Autodesk Inventor part; units mm, degrees
(part 4 of 7)
  line L2571 (-175.0784, 15.5559) -> (-174.9573, 15.634)
  line L2572 (-174.9573, 15.634) -> (-174.8636, 15.7434)
  line L2573 (-174.8636, 15.7434) -> (-174.7994, 15.9277)
  line L2574 (-174.7994, 15.9277) -> (-174.7854, 16.1223)
  line L2575 (-174.7854, 16.1223) -> (-174.7958, 16.3635)
  line L2576 (-174.7958, 16.3635) -> (-174.8284, 16.6028)
  line L2577 (-174.8284, 16.6028) -> (-173.8558, 16.7629)
  line L2578 (-173.8558, 16.7629) -> (-173.7931, 16.4252)
  line L2579 (-173.7931, 16.4252) -> (-173.7637, 16.0838)
  line L2580 (-173.7637, 16.0838) -> (-173.7676, 15.7411)
  line L2581 (-173.7676, 15.7411) -> (-173.805, 15.3997)
  line L2582 (-173.805, 15.3997) -> (-173.8689, 15.171)
  line L2583 (-173.8689, 15.171) -> (-173.9746, 14.9609)
  line L2584 (-173.9746, 14.9609) -> (-174.1185, 14.7748)
  line L2585 (-174.1185, 14.7748) -> (-174.2972, 14.6184)
  line L2586 (-174.2972, 14.6184) -> (-174.4447, 14.5464)
  line L2587 (-174.4447, 14.5464) -> (-174.5992, 14.4921)
  line L2588 (-174.5992, 14.4921) -> (-174.7588, 14.4561)
  line L2589 (-174.7588, 14.4561) -> (-174.9222, 14.4387)
  line L2590 (-174.9222, 14.4387) -> (-175.2129, 14.4186)
  line L2591 (-175.2129, 14.4186) -> (-175.5042, 14.4075)
  line L2592 (-175.5042, 14.4075) -> (-179.4729, 14.4075)
  line L2593 (-179.4729, 14.4075) -> (-179.4729, 13.5989)
  line L2594 (-179.4729, 13.5989) -> (-180.3245, 13.5989)
  line L2595 (-180.3245, 13.5989) -> (-180.3245, 14.4075)
  line L2596 (-180.3245, 14.4075) -> (-181.93, 14.4075)
  line L2597 (-181.93, 14.4075) -> (-182.5901, 15.4973)
  line L2598 (-182.5901, 15.4973) -> (-180.3245, 15.4973)
  line L2599 (-173.844, -41.0652) -> (-173.844, -42.1668)
  line L2600 (-173.844, -42.1668) -> (-180.3245, -42.1668)
  line L2601 (-180.3245, -42.1668) -> (-180.3245, -41.0652)
  line L2602 (-180.3245, -41.0652) -> (-173.844, -41.0652)
  line L2603 (-173.844, -38.3464) -> (-173.844, -39.4441)
  line L2604 (-173.844, -39.4441) -> (-182.7933, -39.4441)
  line L2605 (-182.7933, -39.4441) -> (-182.7933, -38.3464)
  line L2606 (-182.7933, -38.3464) -> (-173.844, -38.3464)
  line L2607 (-179.5823, -48.073) -> (-179.7843, -47.8837)
  line L2608 (-179.7843, -47.8837) -> (-179.964, -47.674)
  line L2609 (-179.964, -47.674) -> (-180.1198, -47.4461)
  line L2610 (-180.1198, -47.4461) -> (-180.2503, -47.2019)
  line L2611 (-180.2503, -47.2019) -> (-180.3496, -46.9447)
  line L2612 (-180.3496, -46.9447) -> (-180.4202, -46.6789)
  line L2613 (-180.4202, -46.6789) -> (-180.4614, -46.4071)
  line L2614 (-180.4614, -46.4071) -> (-180.4729, -46.1316)
  line L2615 (-180.4729, -46.1316) -> (-180.4545, -45.7939)
  line L2616 (-180.4545, -45.7939) -> (-180.4026, -45.4597)
  line L2617 (-180.4026, -45.4597) -> (-180.3417, -45.2394)
  line L2618 (-180.3417, -45.2394) -> (-180.2591, -45.0268)
  line L2619 (-180.2591, -45.0268) -> (-180.1555, -44.8237)
  line L2620 (-180.1555, -44.8237) -> (-180.0315, -44.6316)
  line L2621 (-180.0315, -44.6316) -> (-179.9006, -44.4735)
  line L2622 (-179.9006, -44.4735) -> (-179.7507, -44.3344)
  line L2623 (-179.7507, -44.3344) -> (-179.5841, -44.216)
  line L2624 (-179.5841, -44.216) -> (-179.4026, -44.1199)
  line L2625 (-179.4026, -44.1199) -> (-179.0103, -43.9893)
  line L2626 (-179.0103, -43.9893) -> (-178.6019, -43.9246)
  line L2627 (-178.6019, -43.9246) -> (-178.3932, -43.9046)
  line L2628 (-178.3932, -43.9046) -> (-178.1839, -43.8933)
  line L2629 (-178.1839, -43.8933) -> (-173.844, -43.8933)
  line L2630 (-173.844, -43.8933) -> (-173.844, -44.991)
  line L2631 (-173.844, -44.991) -> (-177.9534, -44.991)
  line L2632 (-177.9534, -44.991) -> (-178.2064, -44.9949)
  line L2633 (-178.2064, -44.9949) -> (-178.456, -45.0299)
  line L2634 (-178.456, -45.0299) -> (-178.6994, -45.0951)
  line L2635 (-178.6994, -45.0951) -> (-178.9339, -45.1902)
  line L2636 (-178.9339, -45.1902) -> (-179.0477, -45.262)
  line L2637 (-179.0477, -45.262) -> (-179.1526, -45.3464)
  line L2638 (-179.1526, -45.3464) -> (-179.3167, -45.5457)
  line L2639 (-179.3167, -45.5457) -> (-179.4339, -45.78)
  line L2640 (-179.4339, -45.78) -> (-179.5042, -46.0496)
  line L2641 (-179.5042, -46.0496) -> (-179.5275, -46.3227)
  line L2642 (-179.5275, -46.3227) -> (-179.512, -46.5964)
  line L2643 (-179.512, -46.5964) -> (-179.4618, -46.8331)
  line L2644 (-179.4618, -46.8331) -> (-179.3818, -47.0603)
  line L2645 (-179.3818, -47.0603) -> (-179.2731, -47.2753)
  line L2646 (-179.2731, -47.2753) -> (-179.137, -47.4753)
  line L2647 (-179.137, -47.4753) -> (-178.9754, -47.6411)
  line L2648 (-178.9754, -47.6411) -> (-178.7933, -47.7839)
  line L2649 (-178.7933, -47.7839) -> (-178.4433, -47.939)
  line L2650 (-178.4433, -47.939) -> (-178.0706, -48.0261)
  line L2651 (-178.0706, -48.0261) -> (-177.7316, -48.0626)
  line L2652 (-177.7316, -48.0626) -> (-177.3909, -48.073)
  line L2653 (-177.3909, -48.073) -> (-173.844, -48.073)
  line L2654 (-173.844, -48.073) -> (-173.844, -49.1707)
  line L2655 (-173.844, -49.1707) -> (-182.7933, -49.1707)
  line L2656 (-182.7933, -49.1707) -> (-182.7933, -48.073)
  line L2657 (-182.7933, -48.073) -> (-179.5823, -48.073)
  line L2658 (-180.4651, 4.47) -> (-180.4377, 4.7226)
  line L2659 (-180.4377, 4.7226) -> (-180.3791, 4.9689)
  line L2660 (-180.3791, 4.9689) -> (-180.2903, 5.2059)
  line L2661 (-180.2903, 5.2059) -> (-180.1722, 5.4309)
  line L2662 (-180.1722, 5.4309) -> (-179.9946, 5.661)
  line L2663 (-179.9946, 5.661) -> (-179.7797, 5.8532)
  line L2664 (-179.7797, 5.8532) -> (-179.5336, 6.0032)
  line L2665 (-179.5336, 6.0032) -> (-179.262, 6.1067)
  line L2666 (-179.262, 6.1067) -> (-179.0241, 6.167)
  line L2667 (-179.0241, 6.167) -> (-178.7826, 6.2087)
  line L2668 (-178.7826, 6.2087) -> (-178.5386, 6.2316)
  line L2669 (-178.5386, 6.2316) -> (-178.2933, 6.2356)
  line L2670 (-178.2933, 6.2356) -> (-173.844, 6.2356)
  line L2671 (-173.844, 6.2356) -> (-173.844, 5.1458)
  line L2672 (-173.844, 5.1458) -> (-177.9261, 5.1458)
  line L2673 (-177.9261, 5.1458) -> (-178.3184, 5.1359)
  line L2674 (-178.3184, 5.1359) -> (-178.7073, 5.0833)
  line L2675 (-178.7073, 5.0833) -> (-178.899, 5.0286)
  line L2676 (-178.899, 5.0286) -> (-179.0727, 4.9355)
  line L2677 (-179.0727, 4.9355) -> (-179.223, 4.808)
  line L2678 (-179.223, 4.808) -> (-179.344, 4.6497)
  line L2679 (-179.344, 4.6497) -> (-179.4364, 4.456)
  line L2680 (-179.4364, 4.456) -> (-179.4957, 4.2513)
  line L2681 (-179.4957, 4.2513) -> (-179.5212, 4.0398)
  line L2682 (-179.5212, 4.0398) -> (-179.512, 3.8254)
  line L2683 (-179.512, 3.8254) -> (-179.4814, 3.6006)
  line L2684 (-179.4814, 3.6006) -> (-179.4175, 3.3871)
  line L2685 (-179.4175, 3.3871) -> (-179.3228, 3.1881)
  line L2686 (-179.3228, 3.1881) -> (-179.1998, 3.0065)
  line L2687 (-179.1998, 3.0065) -> (-179.0509, 2.8455)
  line L2688 (-179.0509, 2.8455) -> (-178.8784, 2.7082)
  line L2689 (-178.8784, 2.7082) -> (-178.685, 2.5976)
  line L2690 (-178.685, 2.5976) -> (-178.4729, 2.5168)
  line L2691 (-178.4729, 2.5168) -> (-178.0457, 2.427)
  line L2692 (-178.0457, 2.427) -> (-177.6097, 2.4036)
  line L2693 (-177.6097, 2.4036) -> (-173.844, 2.4036)
  line L2694 (-173.844, 2.4036) -> (-173.844, 1.3059)
  line L2695 (-173.844, 1.3059) -> (-178.055, 1.3059)
  line L2696 (-178.055, 1.3059) -> (-178.3774, 1.2926)
  line L2697 (-178.3774, 1.2926) -> (-178.6956, 1.2395)
  line L2698 (-178.6956, 1.2395) -> (-178.9495, 1.1536)
  line L2699 (-178.9495, 1.1536) -> (-179.1526, 1.0364)
  line L2700 (-179.1526, 1.0364) -> (-179.283, 0.9168)
  line L2701 (-179.283, 0.9168) -> (-179.3855, 0.7748)
  line L2702 (-179.3855, 0.7748) -> (-179.4576, 0.6152)
  line L2703 (-179.4576, 0.6152) -> (-179.4964, 0.4426)
  line L2704 (-179.4964, 0.4426) -> (-179.5196, 0.088)
  line L2705 (-179.5196, 0.088) -> (-179.4659, -0.259)
  line L2706 (-179.4659, -0.259) -> (-179.3386, -0.5863)
  line L2707 (-179.3386, -0.5863) -> (-179.1409, -0.8816)
  line L2708 (-179.1409, -0.8816) -> (-179.0146, -1.0038)
  line L2709 (-179.0146, -1.0038) -> (-178.8751, -1.1096)
  line L2710 (-178.8751, -1.1096) -> (-178.724, -1.1982)
  line L2711 (-178.724, -1.1982) -> (-178.5628, -1.2683)
  line L2712 (-178.5628, -1.2683) -> (-178.0997, -1.384)
  line L2713 (-178.0997, -1.384) -> (-177.6253, -1.4363)
  line L2714 (-177.6253, -1.4363) -> (-177.2073, -1.448)
  line L2715 (-177.2073, -1.448) -> (-173.844, -1.448)
  line L2716 (-173.844, -1.448) -> (-173.844, -2.5457)
  line L2717 (-173.844, -2.5457) -> (-180.3245, -2.5457)
  line L2718 (-180.3245, -2.5457) -> (-180.3245, -1.5613)
  line L2719 (-180.3245, -1.5613) -> (-179.4183, -1.5613)
  line L2720 (-179.4183, -1.5613) -> (-179.6251, -1.4136)
  line L2721 (-179.6251, -1.4136) -> (-179.8124, -1.2453)
  line L2722 (-179.8124, -1.2453) -> (-179.9787, -1.0583)
  line L2723 (-179.9787, -1.0583) -> (-180.123, -0.8546)
  line L2724 (-180.123, -0.8546) -> (-180.2438, -0.6362)
  line L2725 (-180.2438, -0.6362) -> (-180.34, -0.4051)
  line L2726 (-180.34, -0.4051) -> (-180.4103, -0.1633)
  line L2727 (-180.4103, -0.1633) -> (-180.4534, 0.0872)
  line L2728 (-180.4534, 0.0872) -> (-180.4717, 0.3305)
  line L2729 (-180.4717, 0.3305) -> (-180.4686, 0.5739)
  line L2730 (-180.4686, 0.5739) -> (-180.4443, 0.8162)
  line L2731 (-180.4443, 0.8162) -> (-180.3987, 1.0559)
  line L2732 (-180.3987, 1.0559) -> (-180.305, 1.3372)
  line L2733 (-180.305, 1.3372) -> (-180.213, 1.5188)
  line L2734 (-180.213, 1.5188) -> (-180.1001, 1.6874)
  line L2735 (-180.1001, 1.6874) -> (-179.9675, 1.8409)
  line L2736 (-179.9675, 1.8409) -> (-179.8167, 1.9778)
  line L2737 (-179.8167, 1.9778) -> (-179.5867, 2.1241)
  line L2738 (-179.5867, 2.1241) -> (-179.3362, 2.2317)
  line L2739 (-179.3362, 2.2317) -> (-179.5865, 2.4154)
  line L2740 (-179.5865, 2.4154) -> (-179.8132, 2.6259)
  line L2741 (-179.8132, 2.6259) -> (-180.0144, 2.861)
  line L2742 (-180.0144, 2.861) -> (-180.1878, 3.1184)
  line L2743 (-180.1878, 3.1184) -> (-180.2864, 3.3111)
  line L2744 (-180.2864, 3.3111) -> (-180.364, 3.5125)
  line L2745 (-180.364, 3.5125) -> (-180.4198, 3.721)
  line L2746 (-180.4198, 3.721) -> (-180.4534, 3.9348)
  line L2747 (-180.4534, 3.9348) -> (-180.4724, 4.2021)
  line L2748 (-180.4724, 4.2021) -> (-180.4651, 4.47)
  line L2749 (-182.7854, -53.6121) -> (-182.7482, -52.9791)
  line L2750 (-182.7482, -52.9791) -> (-182.6409, -52.3543)
  line L2751 (-182.6409, -52.3543) -> (-182.5792, -52.146)
  line L2752 (-182.5792, -52.146) -> (-182.4996, -51.9443)
  line L2753 (-182.4996, -51.9443) -> (-182.4029, -51.7503)
  line L2754 (-182.4029, -51.7503) -> (-182.2894, -51.5652)
  line L2755 (-182.2894, -51.5652) -> (-182.0536, -51.2911)
  line L2756 (-182.0536, -51.2911) -> (-181.7801, -51.0579)
  line L2757 (-181.7801, -51.0579) -> (-181.4742, -50.8694)
  line L2758 (-181.4742, -50.8694) -> (-181.1409, -50.7293)
  line L2759 (-181.1409, -50.7293) -> (-180.8639, -50.6516)
  line L2760 (-180.8639, -50.6516) -> (-180.5826, -50.6009)
  line L2761 (-180.5826, -50.6009) -> (-180.2991, -50.5772)
  line L2762 (-180.2991, -50.5772) -> (-180.0153, -50.5802)
  line L2763 (-180.0153, -50.5802) -> (-179.733, -50.6099)
  line L2764 (-179.733, -50.6099) -> (-179.4541, -50.6663)
  line L2765 (-179.4541, -50.6663) -> (-179.1806, -50.749)
  line L2766 (-179.1806, -50.749) -> (-178.9144, -50.8582)
  line L2767 (-178.9144, -50.8582) -> (-178.6835, -50.9871)
  line L2768 (-178.6835, -50.9871) -> (-178.4675, -51.1383)
  line L2769 (-178.4675, -51.1383) -> (-178.2679, -51.3106)
  line L2770 (-178.2679, -51.3106) -> (-178.0862, -51.5027)
  line L2771 (-178.0862, -51.5027) -> (-177.9551, -51.6922)
  line L2772 (-177.9551, -51.6922) -> (-177.8432, -51.8931)
  line L2773 (-177.8432, -51.8931) -> (-177.7513, -52.1038)
  line L2774 (-177.7513, -52.1038) -> (-177.68, -52.323)
  line L2775 (-177.68, -52.323) -> (-177.5868, -52.7182)
  line L2776 (-177.5868, -52.7182) -> (-177.5224, -53.1185)
  line L2777 (-177.5224, -53.1185) -> (-177.487, -53.5225)
  line L2778 (-177.487, -53.5225) -> (-177.4808, -53.9285)
  line L2779 (-177.4808, -53.9285) -> (-177.4808, -56.2214)
  line L2780 (-177.4808, -56.2214) -> (-173.844, -56.2214)
  line L2781 (-173.844, -56.2214) -> (-173.844, -57.405)
  line L2782 (-173.844, -57.405) -> (-182.7933, -57.405)
  line L2783 (-182.7933, -57.405) -> (-182.7933, -54.03)
  line L2784 (-182.7933, -54.03) -> (-182.7854, -53.6121)
  line L2785 (-173.844, -6.9402) -> (-173.844, -8.0418)
  line L2786 (-173.844, -8.0418) -> (-180.3245, -8.0418)
  line L2787 (-180.3245, -8.0418) -> (-180.3245, -6.9402)
  line L2788 (-180.3245, -6.9402) -> (-173.844, -6.9402)
  line L2789 (-173.844, -4.2214) -> (-173.844, -5.3191)
  line L2790 (-173.844, -5.3191) -> (-182.7933, -5.3191)
  line L2791 (-182.7933, -5.3191) -> (-182.7933, -4.2214)
  line L2792 (-182.7933, -4.2214) -> (-173.844, -4.2214)
  line L2793 (-173.844, -35.5652) -> (-173.844, -36.6668)
  line L2794 (-173.844, -36.6668) -> (-180.3245, -36.6668)
  line L2795 (-180.3245, -36.6668) -> (-180.3245, -35.5652)
  line L2796 (-180.3245, -35.5652) -> (-173.844, -35.5652)
  line L2797 (-180.4495, 44.1145) -> (-180.3987, 44.3381)
  line L2798 (-180.3987, 44.3381) -> (-180.326, 44.555)
  line L2799 (-180.326, 44.555) -> (-180.232, 44.7635)
  line L2800 (-180.232, 44.7635) -> (-180.1175, 44.9621)
  line L2801 (-180.1175, 44.9621) -> (-179.0979, 44.5871)
  line L2802 (-179.0979, 44.5871) -> (-179.2175, 44.3584)
  line L2803 (-179.2175, 44.3584) -> (-179.2959, 44.1144)
  line L2804 (-179.2959, 44.1144) -> (-179.332, 43.8607)
  line L2805 (-179.332, 43.8607) -> (-179.3245, 43.6028)
  line L2806 (-179.3245, 43.6028) -> (-179.2233, 43.3038)
  line L2807 (-179.2233, 43.3038) -> (-179.0473, 43.0488)
  line L2808 (-179.0473, 43.0488) -> (-178.8087, 42.851)
  line L2809 (-178.8087, 42.851) -> (-178.5198, 42.7239)
  line L2810 (-178.5198, 42.7239) -> (-178.2054, 42.6419)
  line L2811 (-178.2054, 42.6419) -> (-177.8861, 42.5838)
  line L2812 (-177.8861, 42.5838) -> (-177.5634, 42.5499)
  line L2813 (-177.5634, 42.5499) -> (-177.2386, 42.5403)
  line L2814 (-177.2386, 42.5403) -> (-173.844, 42.5403)
  line L2815 (-173.844, 42.5403) -> (-173.844, 41.4426)
  line L2816 (-173.844, 41.4426) -> (-180.3245, 41.4426)
  line L2817 (-180.3245, 41.4426) -> (-180.3245, 42.4309)
  line L2818 (-180.3245, 42.4309) -> (-179.344, 42.4309)
  line L2819 (-179.344, 42.4309) -> (-179.7479, 42.671)
  line L2820 (-179.7479, 42.671) -> (-180.1136, 42.9661)
  line L2821 (-180.1136, 42.9661) -> (-180.2676, 43.1524)
  line L2822 (-180.2676, 43.1524) -> (-180.3807, 43.3634)
  line L2823 (-180.3807, 43.3634) -> (-180.4501, 43.5926)
  line L2824 (-180.4501, 43.5926) -> (-180.4729, 43.8332)
  line L2825 (-180.4729, 43.8332) -> (-180.4495, 44.1145)
  line L2826 (-181.7347, -9.7878) -> (-181.7347, -15.073)
  line L2827 (-181.7347, -15.073) -> (-178.9964, -15.073)
  line L2828 (-178.9964, -15.073) -> (-178.9964, -10.1238)
  line L2829 (-178.9964, -10.1238) -> (-177.9456, -10.1238)
  line L2830 (-177.9456, -10.1238) -> (-177.9456, -15.073)
  line L2831 (-177.9456, -15.073) -> (-174.8987, -15.073)
  line L2832 (-174.8987, -15.073) -> (-174.8987, -9.5808)
  line L2833 (-174.8987, -9.5808) -> (-173.844, -9.5808)
  line L2834 (-173.844, -9.5808) -> (-173.844, -16.2566)
  line L2835 (-173.844, -16.2566) -> (-182.7933, -16.2566)
  line L2836 (-182.7933, -16.2566) -> (-182.7933, -9.7878)
  line L2837 (-182.7933, -9.7878) -> (-181.7347, -9.7878)
  line L2838 (-180.4612, 30.7942) -> (-180.4125, 31.1189)
  line L2839 (-180.4125, 31.1189) -> (-180.3217, 31.433)
  line L2840 (-180.3217, 31.433) -> (-180.1903, 31.7323)
  line L2841 (-180.1903, 31.7323) -> (-180.0198, 32.0129)
  line L2842 (-180.0198, 32.0129) -> (-179.8765, 32.1752)
  line L2843 (-179.8765, 32.1752) -> (-179.7132, 32.3158)
  line L2844 (-179.7132, 32.3158) -> (-179.5323, 32.4329)
  line L2845 (-179.5323, 32.4329) -> (-179.3362, 32.5246)
  line L2846 (-179.3362, 32.5246) -> (-179.129, 32.6018)
  line L2847 (-179.129, 32.6018) -> (-178.9156, 32.6576)
  line L2848 (-178.9156, 32.6576) -> (-178.6976, 32.6919)
  line L2849 (-178.6976, 32.6919) -> (-178.4769, 32.7043)
  line L2850 (-178.4769, 32.7043) -> (-178.1528, 32.7168)
  line L2851 (-178.1528, 32.7168) -> (-177.8284, 32.72)
  line L2852 (-177.8284, 32.72) -> (-173.844, 32.72)
  line L2853 (-173.844, 32.72) -> (-173.844, 31.6223)
  line L2854 (-173.844, 31.6223) -> (-177.7854, 31.6223)
  line L2855 (-177.7854, 31.6223) -> (-178.1957, 31.6106)
  line L2856 (-178.1957, 31.6106) -> (-178.6019, 31.552)
  line L2857 (-178.6019, 31.552) -> (-178.8645, 31.4628)
  line L2858 (-178.8645, 31.4628) -> (-179.0935, 31.3136)
  line L2859 (-179.0935, 31.3136) -> (-179.2788, 31.1126)
  line L2860 (-179.2788, 31.1126) -> (-179.4104, 30.8684)
  line L2861 (-179.4104, 30.8684) -> (-179.4939, 30.5768)
  line L2862 (-179.4939, 30.5768) -> (-179.5198, 30.2746)
  line L2863 (-179.5198, 30.2746) -> (-179.4925, 29.9348)
  line L2864 (-179.4925, 29.9348) -> (-179.4104, 29.6184)
  line L2865 (-179.4104, 29.6184) -> (-179.2698, 29.3293)
  line L2866 (-179.2698, 29.3293) -> (-179.0745, 29.0637)
  line L2867 (-179.0745, 29.0637) -> (-178.9347, 28.9349)
  line L2868 (-178.9347, 28.9349) -> (-178.7791, 28.8271)
  line L2869 (-178.7791, 28.8271) -> (-178.6101, 28.742)
  line L2870 (-178.6101, 28.742) -> (-178.43, 28.6809)
  line L2871 (-178.43, 28.6809) -> (-178.1724, 28.6197)
  line L2872 (-178.1724, 28.6197) -> (-177.9113, 28.5777)
  line L2873 (-177.9113, 28.5777) -> (-177.6479, 28.5551)
  line L2874 (-177.6479, 28.5551) -> (-177.3831, 28.552)
  line L2875 (-177.3831, 28.552) -> (-173.844, 28.552)
  line L2876 (-173.844, 28.552) -> (-173.844, 27.4543)
  line L2877 (-173.844, 27.4543) -> (-180.3245, 27.4543)
  line L2878 (-180.3245, 27.4543) -> (-180.3245, 28.4426)
  line L2879 (-180.3245, 28.4426) -> (-179.4026, 28.4426)
  line L2880 (-179.4026, 28.4426) -> (-179.6445, 28.6215)
  line L2881 (-179.6445, 28.6215) -> (-179.8608, 28.8288)
  line L2882 (-179.8608, 28.8288) -> (-180.0492, 29.0617)
  line L2883 (-180.0492, 29.0617) -> (-180.2073, 29.3176)
  line L2884 (-180.2073, 29.3176) -> (-180.327, 29.6009)
  line L2885 (-180.327, 29.6009) -> (-180.4116, 29.8954)
  line L2886 (-180.4116, 29.8954) -> (-180.4605, 30.1979)
  line L2887 (-180.4605, 30.1979) -> (-180.4729, 30.5051)
  line L2888 (-180.4729, 30.5051) -> (-180.4612, 30.7942)
  line L2889 (-173.844, 25.8098) -> (-173.844, 24.7121)
  line L2890 (-173.844, 24.7121) -> (-180.3245, 24.7121)
  line L2891 (-180.3245, 24.7121) -> (-180.3245, 25.8098)
  line L2892 (-180.3245, 25.8098) -> (-173.844, 25.8098)
  line L2893 (-179.6019, -24.3152) -> (-179.5417, -24.5783)
  line L2894 (-179.5417, -24.5783) -> (-179.4377, -24.8252)
  line L2895 (-179.4377, -24.8252) -> (-179.2927, -25.0505)
  line L2896 (-179.2927, -25.0505) -> (-179.1097, -25.2488)
  line L2897 (-179.1097, -25.2488) -> (-178.8983, -25.4302)
  line L2898 (-178.8983, -25.4302) -> (-178.6663, -25.5823)
  line L2899 (-178.6663, -25.5823) -> (-178.4168, -25.7034)
  line L2900 (-178.4168, -25.7034) -> (-178.1526, -25.7918)
  line L2901 (-178.1526, -25.7918) -> (-177.608, -25.8918)
  line L2902 (-177.608, -25.8918) -> (-177.0574, -25.9265)
  line L2903 (-177.0574, -25.9265) -> (-176.5065, -25.8958)
  line L2904 (-176.5065, -25.8958) -> (-175.9612, -25.7996)
  line L2905 (-175.9612, -25.7996) -> (-175.6269, -25.6864)
  line L2906 (-175.6269, -25.6864) -> (-175.3227, -25.5135)
  line L2907 (-175.3227, -25.5135) -> (-175.0565, -25.2863)
  line L2908 (-175.0565, -25.2863) -> (-174.8362, -25.0105)
  line L2909 (-174.8362, -25.0105) -> (-174.7131, -24.7698)
  line L2910 (-174.7131, -24.7698) -> (-174.635, -24.5173)
  line L2911 (-174.635, -24.5173) -> (-174.6014, -24.2586)
  line L2912 (-174.6014, -24.2586) -> (-174.6114, -23.9994)
  line L2913 (-174.6114, -23.9994) -> (-174.6645, -23.7456)
  line L2914 (-174.6645, -23.7456) -> (-174.7598, -23.5027)
  line L2915 (-174.7598, -23.5027) -> (-174.8967, -23.2766)
  line L2916 (-174.8967, -23.2766) -> (-175.0745, -23.073)
  line L2917 (-175.0745, -23.073) -> (-175.2797, -22.8949)
  line L2918 (-175.2797, -22.8949) -> (-175.5058, -22.7464)
  line L2919 (-175.5058, -22.7464) -> (-175.7496, -22.6294)
  line L2920 (-175.7496, -22.6294) -> (-176.0081, -22.5457)
  line L2921 (-176.0081, -22.5457) -> (-176.5589, -22.4474)
  line L2922 (-176.5589, -22.4474) -> (-177.1155, -22.4146)
  line L2923 (-177.1155, -22.4146) -> (-177.6721, -22.4474)
  line L2924 (-177.6721, -22.4474) -> (-178.2229, -22.5457)
  line L2925 (-178.2229, -22.5457) -> (-178.5619, -22.6593)
  line L2926 (-178.5619, -22.6593) -> (-178.8714, -22.8322)
  line L2927 (-178.8714, -22.8322) -> (-179.1438, -23.0591)
  line L2928 (-179.1438, -23.0591) -> (-179.3714, -23.3347)
  line L2929 (-179.3714, -23.3347) -> (-179.4939, -23.5615)
  line L2930 (-179.4939, -23.5615) -> (-179.5741, -23.8044)
  line L2931 (-179.5741, -23.8044) -> (-179.6106, -24.0576)
  line L2932 (-179.6106, -24.0576) -> (-179.6019, -24.3152)
  line L2933 (-179.6019, -31.3152) -> (-179.5417, -31.5783)
  line L2934 (-179.5417, -31.5783) -> (-179.4377, -31.8252)
  line L2935 (-179.4377, -31.8252) -> (-179.2927, -32.0505)
  line L2936 (-179.2927, -32.0505) -> (-179.1097, -32.2488)
  line L2937 (-179.1097, -32.2488) -> (-178.8983, -32.4302)
  line L2938 (-178.8983, -32.4302) -> (-178.6663, -32.5823)
  line L2939 (-178.6663, -32.5823) -> (-178.4168, -32.7034)
  line L2940 (-178.4168, -32.7034) -> (-178.1526, -32.7918)
  line L2941 (-178.1526, -32.7918) -> (-177.608, -32.8918)
  line L2942 (-177.608, -32.8918) -> (-177.0574, -32.9265)
  line L2943 (-177.0574, -32.9265) -> (-176.5065, -32.8958)
  line L2944 (-176.5065, -32.8958) -> (-175.9612, -32.7996)
  line L2945 (-175.9612, -32.7996) -> (-175.6269, -32.6864)
  line L2946 (-175.6269, -32.6864) -> (-175.3227, -32.5135)
  line L2947 (-175.3227, -32.5135) -> (-175.0565, -32.2863)
  line L2948 (-175.0565, -32.2863) -> (-174.8362, -32.0105)
  line L2949 (-174.8362, -32.0105) -> (-174.7131, -31.7698)
  line L2950 (-174.7131, -31.7698) -> (-174.635, -31.5173)
  line L2951 (-174.635, -31.5173) -> (-174.6014, -31.2586)
  line L2952 (-174.6014, -31.2586) -> (-174.6114, -30.9994)
  line L2953 (-174.6114, -30.9994) -> (-174.6645, -30.7456)
  line L2954 (-174.6645, -30.7456) -> (-174.7598, -30.5027)
  line L2955 (-174.7598, -30.5027) -> (-174.8967, -30.2766)
  line L2956 (-174.8967, -30.2766) -> (-175.0745, -30.073)
  line L2957 (-175.0745, -30.073) -> (-175.2797, -29.8949)
  line L2958 (-175.2797, -29.8949) -> (-175.5058, -29.7464)
  line L2959 (-175.5058, -29.7464) -> (-175.7496, -29.6294)
  line L2960 (-175.7496, -29.6294) -> (-176.0081, -29.5457)
  line L2961 (-176.0081, -29.5457) -> (-176.5589, -29.4474)
  line L2962 (-176.5589, -29.4474) -> (-177.1155, -29.4146)
  line L2963 (-177.1155, -29.4146) -> (-177.6721, -29.4474)
  line L2964 (-177.6721, -29.4474) -> (-178.2229, -29.5457)
  line L2965 (-178.2229, -29.5457) -> (-178.5619, -29.6593)
  line L2966 (-178.5619, -29.6593) -> (-178.8714, -29.8322)
  line L2967 (-178.8714, -29.8322) -> (-179.1438, -30.0591)
  line L2968 (-179.1438, -30.0591) -> (-179.3714, -30.3347)
  line L2969 (-179.3714, -30.3347) -> (-179.4939, -30.5615)
  line L2970 (-179.4939, -30.5615) -> (-179.5741, -30.8044)
  line L2971 (-179.5741, -30.8044) -> (-179.6106, -31.0576)
  line L2972 (-179.6106, -31.0576) -> (-179.6019, -31.3152)
  line L2973 (-179.5628, 36.9426) -> (-179.5184, 36.6758)
  line L2974 (-179.5184, 36.6758) -> (-179.436, 36.4229)
  line L2975 (-179.436, 36.4229) -> (-179.3182, 36.1876)
  line L2976 (-179.3182, 36.1876) -> (-179.168, 35.973)
  line L2977 (-179.168, 35.973) -> (-178.9879, 35.7828)
  line L2978 (-178.9879, 35.7828) -> (-178.7809, 35.6202)
  line L2979 (-178.7809, 35.6202) -> (-178.5497, 35.4888)
  line L2980 (-178.5497, 35.4888) -> (-178.2972, 35.3918)
  line L2981 (-178.2972, 35.3918) -> (-178.0053, 35.3209)
  line L2982 (-178.0053, 35.3209) -> (-177.7073, 35.2825)
  line L2983 (-177.7073, 35.2825) -> (-177.7073, 38.9036)
  line L2984 (-177.7073, 38.9036) -> (-178.0686, 38.8532)
  line L2985 (-178.0686, 38.8532) -> (-178.4222, 38.7629)
  line L2986 (-178.4222, 38.7629) -> (-178.7034, 38.6418)
  line L2987 (-178.7034, 38.6418) -> (-178.9339, 38.4895)
  line L2988 (-178.9339, 38.4895) -> (-179.2086, 38.2111)
  line L2989 (-179.2086, 38.2111) -> (-179.4106, 37.8819)
  line L2990 (-179.4106, 37.8819) -> (-179.5335, 37.5156)
  line L2991 (-179.5335, 37.5156) -> (-179.5706, 37.1262)
  line L2992 (-179.5706, 37.1262) -> (-179.5628, 36.9426)
  line L2993 (-179.5628, 20.1926) -> (-179.5184, 19.9258)
  line L2994 (-179.5184, 19.9258) -> (-179.436, 19.6729)
  line L2995 (-179.436, 19.6729) -> (-179.3182, 19.4376)
  line L2996 (-179.3182, 19.4376) -> (-179.168, 19.223)
  line L2997 (-179.168, 19.223) -> (-178.9879, 19.0328)
  line L2998 (-178.9879, 19.0328) -> (-178.7809, 18.8702)
  line L2999 (-178.7809, 18.8702) -> (-178.5497, 18.7388)
  line L3000 (-178.5497, 18.7388) -> (-178.2972, 18.6418)
  line L3001 (-178.2972, 18.6418) -> (-178.0053, 18.5709)
  line L3002 (-178.0053, 18.5709) -> (-177.7073, 18.5325)
  line L3003 (-177.7073, 18.5325) -> (-177.7073, 22.1536)
  line L3004 (-177.7073, 22.1536) -> (-178.0686, 22.1032)
  line L3005 (-178.0686, 22.1032) -> (-178.4222, 22.0129)
  line L3006 (-178.4222, 22.0129) -> (-178.7034, 21.8918)
  line L3007 (-178.7034, 21.8918) -> (-178.9339, 21.7395)
  line L3008 (-178.9339, 21.7395) -> (-179.2086, 21.4611)
  line L3009 (-179.2086, 21.4611) -> (-179.4106, 21.1318)
  line L3010 (-179.4106, 21.1318) -> (-179.5335, 20.7656)
  line L3011 (-179.5335, 20.7656) -> (-179.5706, 20.3762)
  line L3012 (-179.5706, 20.3762) -> (-179.5628, 20.1926)
  line L3013 (-181.7347, -56.2214) -> (-178.5394, -56.2214)
  line L3014 (-178.5394, -56.2214) -> (-178.5394, -53.9089)
  line L3015 (-178.5394, -53.9089) -> (-178.5413, -53.6104)
  line L3016 (-178.5413, -53.6104) -> (-178.5695, -53.3138)
  line L3017 (-178.5695, -53.3138) -> (-178.6236, -53.0208)
  line L3018 (-178.6236, -53.0208) -> (-178.7034, -52.7332)
  line L3019 (-178.7034, -52.7332) -> (-178.778, -52.5585)
  line L3020 (-178.778, -52.5585) -> (-178.8746, -52.398)
  line L3021 (-178.8746, -52.398) -> (-178.991, -52.2534)
  line L3022 (-178.991, -52.2534) -> (-179.1254, -52.1263)
  line L3023 (-179.1254, -52.1263) -> (-179.2755, -52.0185)
  line L3024 (-179.2755, -52.0185) -> (-179.4396, -51.9315)
  line L3025 (-179.4396, -51.9315) -> (-179.6154, -51.8671)
  line L3026 (-179.6154, -51.8671) -> (-179.8011, -51.8269)
  line L3027 (-179.8011, -51.8269) -> (-180.0853, -51.7948)
  line L3028 (-180.0853, -51.7948) -> (-180.3695, -51.8059)
  line L3029 (-180.3695, -51.8059) -> (-180.6488, -51.8598)
  line L3030 (-180.6488, -51.8598) -> (-180.9183, -51.9558)
  line L3031 (-180.9183, -51.9558) -> (-181.0749, -52.0423)
  line L3032 (-181.0749, -52.0423) -> (-181.2188, -52.1476)
  line L3033 (-181.2188, -52.1476) -> (-181.3481, -52.2703)
  line L3034 (-181.3481, -52.2703) -> (-181.4612, -52.4089)
  line L3035 (-181.4612, -52.4089) -> (-181.5703, -52.6043)
  line L3036 (-181.5703, -52.6043) -> (-181.6496, -52.8123)
  line L3037 (-181.6496, -52.8123) -> (-181.6982, -53.0296)
  line L3038 (-181.6982, -53.0296) -> (-181.7151, -53.2527)
  line L3039 (-181.7151, -53.2527) -> (-181.7282, -53.4967)
  line L3040 (-181.7282, -53.4967) -> (-181.7347, -53.741)
  line L3041 (-181.7347, -53.741) -> (-181.7347, -56.2214)
  line L3042 (-181.5276, -6.9402) -> (-181.5276, -8.0418)
  line L3043 (-181.5276, -8.0418) -> (-182.7933, -8.0418)
  line L3044 (-182.7933, -8.0418) -> (-182.7933, -6.9402)
  line L3045 (-182.7933, -6.9402) -> (-181.5276, -6.9402)
  line L3046 (-181.5276, -35.5652) -> (-181.5276, -36.6668)
  line L3047 (-181.5276, -36.6668) -> (-182.7933, -36.6668)
  line L3048 (-182.7933, -36.6668) -> (-182.7933, -35.5652)
  line L3049 (-182.7933, -35.5652) -> (-181.5276, -35.5652)
  line L3050 (-181.5276, -41.0652) -> (-181.5276, -42.1668)
  line L3051 (-181.5276, -42.1668) -> (-182.7933, -42.1668)
  line L3052 (-182.7933, -42.1668) -> (-182.7933, -41.0652)
  line L3053 (-182.7933, -41.0652) -> (-181.5276, -41.0652)
  line L3054 (-181.5276, 25.8098) -> (-181.5276, 24.7121)
  line L3055 (-181.5276, 24.7121) -> (-182.7933, 24.7121)
  line L3056 (-182.7933, 24.7121) -> (-182.7933, 25.8098)
  line L3057 (-182.7933, 25.8098) -> (-181.5276, 25.8098)
  line L3058 (-197.3011, -41.7722) -> (-197.2404, -41.3292)
  line L3059 (-197.2404, -41.3292) -> (-197.1409, -40.8933)
  line L3060 (-197.1409, -40.8933) -> (-197.0003, -40.4988)
  line L3061 (-197.0003, -40.4988) -> (-196.8206, -40.1433)
  line L3062 (-196.8206, -40.1433) -> (-196.6019, -39.8269)
  line L3063 (-196.6019, -39.8269) -> (-196.3479, -39.5574)
  line L3064 (-196.3479, -39.5574) -> (-196.055, -39.3308)
  line L3065 (-196.055, -39.3308) -> (-195.7347, -39.1511)
  line L3066 (-195.7347, -39.1511) -> (-195.3909, -39.0183)
  line L3067 (-195.3909, -39.0183) -> (-195.0276, -38.9324)
  line L3068 (-195.0276, -38.9324) -> (-194.6448, -38.8933)
  line L3069 (-194.6448, -38.8933) -> (-194.5589, -40.0261)
  line L3070 (-194.5589, -40.0261) -> (-194.7947, -40.0583)
  line L3071 (-194.7947, -40.0583) -> (-195.0245, -40.1171)
  line L3072 (-195.0245, -40.1171) -> (-195.2461, -40.2016)
  line L3073 (-195.2461, -40.2016) -> (-195.4573, -40.3113)
  line L3074 (-195.4573, -40.3113) -> (-195.7049, -40.5027)
  line L3075 (-195.7049, -40.5027) -> (-195.9094, -40.7359)
  line L3076 (-195.9094, -40.7359) -> (-196.0655, -41.0039)
  line L3077 (-196.0655, -41.0039) -> (-196.1683, -41.2996)
  line L3078 (-196.1683, -41.2996) -> (-196.2566, -41.8035)
  line L3079 (-196.2566, -41.8035) -> (-196.2781, -42.3124)
  line L3080 (-196.2781, -42.3124) -> (-196.233, -42.8198)
  line L3081 (-196.233, -42.8198) -> (-196.1214, -43.3191)
  line L3082 (-196.1214, -43.3191) -> (-195.9992, -43.5995)
  line L3083 (-195.9992, -43.5995) -> (-195.8215, -43.8442)
  line L3084 (-195.8215, -43.8442) -> (-195.5955, -44.045)
  line L3085 (-195.5955, -44.045) -> (-195.3284, -44.1941)
  line L3086 (-195.3284, -44.1941) -> (-195.0665, -44.2576)
  line L3087 (-195.0665, -44.2576) -> (-194.8007, -44.2563)
  line L3088 (-194.8007, -44.2563) -> (-194.543, -44.1917)
  line L3089 (-194.543, -44.1917) -> (-194.305, -44.0652)
  line L3090 (-194.305, -44.0652) -> (-194.1409, -43.9168)
  line L3091 (-194.1409, -43.9168) -> (-193.9556, -43.62)
  line L3092 (-193.9556, -43.62) -> (-193.8245, -43.2957)
  line L3093 (-193.8245, -43.2957) -> (-193.601, -42.5457)
  line L3094 (-193.601, -42.5457) -> (-193.4222, -41.7839)
  line L3095 (-193.4222, -41.7839) -> (-193.2312, -41.0329)
  line L3096 (-193.2312, -41.0329) -> (-192.9925, -40.2957)
  line L3097 (-192.9925, -40.2957) -> (-192.93, -40.1472)
  line L3098 (-192.93, -40.1472) -> (-192.7386, -39.7839)
  line L3099 (-192.7386, -39.7839) -> (-192.5237, -39.4714)
  line L3100 (-192.5237, -39.4714) -> (-192.2815, -39.2058)
  line L3101 (-192.2815, -39.2058) -> (-192.0198, -38.9949)
  line L3102 (-192.0198, -38.9949) -> (-191.7308, -38.8308)
  line L3103 (-191.7308, -38.8308) -> (-191.4261, -38.7175)
  line L3104 (-191.4261, -38.7175) -> (-191.0896, -38.6466)
  line L3105 (-191.0896, -38.6466) -> (-190.7464, -38.6238)
  line L3106 (-190.7464, -38.6238) -> (-190.3948, -38.6472)
  line L3107 (-190.3948, -38.6472) -> (-190.0511, -38.7253)
  line L3108 (-190.0511, -38.7253) -> (-189.7229, -38.8543)
  line L3109 (-189.7229, -38.8543) -> (-189.3987, -39.0339)
  line L3110 (-189.3987, -39.0339) -> (-189.1019, -39.2605)
  line L3111 (-189.1019, -39.2605) -> (-188.8401, -39.53)
  line L3112 (-188.8401, -39.53) -> (-188.6097, -39.8464)
  line L3113 (-188.6097, -39.8464) -> (-188.4146, -40.2136)
  line L3114 (-188.4146, -40.2136) -> (-188.262, -40.6003)
  line L3115 (-188.262, -40.6003) -> (-188.1526, -41.0222)
  line L3116 (-188.1526, -41.0222) -> (-188.0731, -41.7104)
  line L3117 (-188.0731, -41.7104) -> (-188.0776, -42.4006)
  line L3118 (-188.0776, -42.4006) -> (-188.1654, -43.0852)
  line L3119 (-188.1654, -43.0852) -> (-188.3362, -43.7566)
  line L3120 (-188.3362, -43.7566) -> (-188.5027, -44.1513)
  line L3121 (-188.5027, -44.1513) -> (-188.7236, -44.5158)
  line L3122 (-188.7236, -44.5158) -> (-188.9949, -44.8444)
  line L3123 (-188.9949, -44.8444) -> (-189.3128, -45.1316)
  line L3124 (-189.3128, -45.1316) -> (-189.4847, -45.2527)
  line L3125 (-189.4847, -45.2527) -> (-189.8519, -45.4597)
  line L3126 (-189.8519, -45.4597) -> (-190.2425, -45.6121)
  line L3127 (-190.2425, -45.6121) -> (-190.6565, -45.7058)
  line L3128 (-190.6565, -45.7058) -> (-191.094, -45.7449)
  line L3129 (-191.094, -45.7449) -> (-191.1917, -44.6277)
  line L3130 (-191.1917, -44.6277) -> (-190.9667, -44.5985)
  line L3131 (-190.9667, -44.5985) -> (-190.7457, -44.5494)
  line L3132 (-190.7457, -44.5494) -> (-190.5299, -44.4809)
  line L3133 (-190.5299, -44.4809) -> (-190.3206, -44.3933)
  line L3134 (-190.3206, -44.3933) -> (-190.1428, -44.297)
  line L3135 (-190.1428, -44.297) -> (-189.9788, -44.1799)
  line L3136 (-189.9788, -44.1799) -> (-189.8304, -44.0436)
  line L3137 (-189.8304, -44.0436) -> (-189.6995, -43.8894)
  line L3138 (-189.6995, -43.8894) -> (-189.5242, -43.6172)
  line L3139 (-189.5242, -43.6172) -> (-189.381, -43.328)
  line L3140 (-189.381, -43.328) -> (-189.2711, -43.0245)
  line L3141 (-189.2711, -43.0245) -> (-189.1956, -42.7097)
  line L3142 (-189.1956, -42.7097) -> (-189.1392, -42.2966)
  line L3143 (-189.1392, -42.2966) -> (-189.1283, -41.881)
  line L3144 (-189.1283, -41.881) -> (-189.1628, -41.4667)
  line L3145 (-189.1628, -41.4667) -> (-189.2425, -41.0574)
  line L3146 (-189.2425, -41.0574) -> (-189.318, -40.8129)
  line L3147 (-189.318, -40.8129) -> (-189.4229, -40.5805)
  line L3148 (-189.4229, -40.5805) -> (-189.5557, -40.363)
  line L3149 (-189.5557, -40.363) -> (-189.7151, -40.1628)
  line L3150 (-189.7151, -40.1628) -> (-189.851, -40.0396)
  line L3151 (-189.851, -40.0396) -> (-190.0006, -39.9382)
  line L3152 (-190.0006, -39.9382) -> (-190.1614, -39.8594)
  line L3153 (-190.1614, -39.8594) -> (-190.3309, -39.8039)
  line L3154 (-190.3309, -39.8039) -> (-190.5064, -39.7722)
  line L3155 (-190.5064, -39.7722) -> (-190.6853, -39.765)
  line L3156 (-190.6853, -39.765) -> (-190.8651, -39.783)
  line L3157 (-190.8651, -39.783) -> (-191.0433, -39.8269)
  line L3158 (-191.0433, -39.8269) -> (-191.2314, -39.9106)
  line L3159 (-191.2314, -39.9106) -> (-191.4013, -40.0244)
  line L3160 (-191.4013, -40.0244) -> (-191.5494, -40.1654)
  line L3161 (-191.5494, -40.1654) -> (-191.6722, -40.3308)
  line L3162 (-191.6722, -40.3308) -> (-191.8072, -40.5837)
  line L3163 (-191.8072, -40.5837) -> (-191.9222, -40.8459)
  line L3164 (-191.9222, -40.8459) -> (-192.0167, -41.1162)
  line L3165 (-192.0167, -41.1162) -> (-192.0901, -41.3933)
  line L3166 (-192.0901, -41.3933) -> (-192.2958, -42.1851)
  line L3167 (-192.2958, -42.1851) -> (-192.4925, -42.9793)
  line L3168 (-192.4925, -42.9793) -> (-192.6707, -43.5677)
  line L3169 (-192.6707, -43.5677) -> (-192.9065, -44.1355)
  line L3170 (-192.9065, -44.1355) -> (-193.0787, -44.4251)
  line L3171 (-193.0787, -44.4251) -> (-193.2815, -44.6941)
  line L3172 (-193.2815, -44.6941) -> (-193.6083, -44.9982)
  line L3173 (-193.6083, -44.9982) -> (-193.9884, -45.2224)
  line L3174 (-193.9884, -45.2224) -> (-194.4077, -45.3602)
  line L3175 (-194.4077, -45.3602) -> (-194.8519, -45.405)
  line L3176 (-194.8519, -45.405) -> (-195.1878, -45.3816)
  line L3177 (-195.1878, -45.3816) -> (-195.5111, -45.3064)
  line L3178 (-195.5111, -45.3064) -> (-195.8206, -45.1863)
  line L3179 (-195.8206, -45.1863) -> (-196.1214, -45.0183)
  line L3180 (-196.1214, -45.0183) -> (-196.3987, -44.8035)
  line L3181 (-196.3987, -44.8035) -> (-196.637, -44.5457)
  line L3182 (-196.637, -44.5457) -> (-196.844, -44.2449)
  line L3183 (-196.844, -44.2449) -> (-197.0186, -43.8909)
  line L3184 (-197.0186, -43.8909) -> (-197.1487, -43.5183)
  line L3185 (-197.1487, -43.5183) -> (-197.2244, -43.2079)
  line L3186 (-197.2244, -43.2079) -> (-197.2783, -42.8934)
  line L3187 (-197.2783, -42.8934) -> (-197.3105, -42.5759)
  line L3188 (-197.3105, -42.5759) -> (-197.3206, -42.2566)
  line L3189 (-197.3206, -42.2566) -> (-197.3011, -41.7722)
  line L3190 (-194.8323, 6.4934) -> (-194.7794, 6.8673)
  line L3191 (-194.7794, 6.8673) -> (-194.6772, 7.2252)
  line L3192 (-194.6772, 7.2252) -> (-194.5286, 7.5631)
  line L3193 (-194.5286, 7.5631) -> (-194.3367, 7.8765)
  line L3194 (-194.3367, 7.8765) -> (-194.1044, 8.1614)
  line L3195 (-194.1044, 8.1614) -> (-193.8348, 8.4134)
  line L3196 (-193.8348, 8.4134) -> (-193.5309, 8.6283)
  line L3197 (-193.5309, 8.6283) -> (-193.1956, 8.802)
  line L3198 (-193.1956, 8.802) -> (-192.8739, 8.9239)
  line L3199 (-192.8739, 8.9239) -> (-192.5434, 9.0169)
  line L3200 (-192.5434, 9.0169) -> (-192.2059, 9.0806)
  line L3201 (-192.2059, 9.0806) -> (-191.8636, 9.1145)
  line L3202 (-191.8636, 9.1145) -> (-191.5218, 9.1235)
  line L3203 (-191.5218, 9.1235) -> (-191.18, 9.1184)
  line L3204 (-191.18, 9.1184) -> (-191.18, 4.2864)
  line L3205 (-191.18, 4.2864) -> (-190.8858, 4.3093)
  line L3206 (-190.8858, 4.3093) -> (-190.5963, 4.3616)
  line L3207 (-190.5963, 4.3616) -> (-190.3134, 4.4426)
  line L3208 (-190.3134, 4.4426) -> (-190.0394, 4.552)
  line L3209 (-190.0394, 4.552) -> (-189.8038, 4.6816)
  line L3210 (-189.8038, 4.6816) -> (-189.5931, 4.8417)
  line L3211 (-189.5931, 4.8417) -> (-189.4096, 5.0286)
  line L3212 (-189.4096, 5.0286) -> (-189.2554, 5.239)
  line L3213 (-189.2554, 5.239) -> (-189.1329, 5.4692)
  line L3214 (-189.1329, 5.4692) -> (-189.0441, 5.7157)
  line L3215 (-189.0441, 5.7157) -> (-188.9913, 5.9749)
  line L3216 (-188.9913, 5.9749) -> (-188.9769, 6.2434)
  line L3217 (-188.9769, 6.2434) -> (-188.9951, 6.5275)
  line L3218 (-188.9951, 6.5275) -> (-189.055, 6.8059)
  line L3219 (-189.055, 6.8059) -> (-189.1523, 7.0514)
  line L3220 (-189.1523, 7.0514) -> (-189.2933, 7.2747)
  line L3221 (-189.2933, 7.2747) -> (-189.4825, 7.4831)
  line L3222 (-189.4825, 7.4831) -> (-189.7034, 7.6575)
  line L3223 (-189.7034, 7.6575) -> (-189.9949, 7.8247)
  line L3224 (-189.9949, 7.8247) -> (-190.305, 7.9543)
  line L3225 (-190.305, 7.9543) -> (-190.1644, 9.0911)
  line L3226 (-190.1644, 9.0911) -> (-189.8262, 8.9825)
  line L3227 (-189.8262, 8.9825) -> (-189.5048, 8.8344)
  line L3228 (-189.5048, 8.8344) -> (-189.2036, 8.6486)
  line L3229 (-189.2036, 8.6486) -> (-188.9261, 8.427)
  line L3230 (-188.9261, 8.427) -> (-188.6508, 8.1266)
  line L3231 (-188.6508, 8.1266) -> (-188.4271, 7.7891)
  line L3232 (-188.4271, 7.7891) -> (-188.2585, 7.4209)
  line L3233 (-188.2585, 7.4209) -> (-188.1487, 7.0286)
  line L3234 (-188.1487, 7.0286) -> (-188.0874, 6.5853)
  line L3235 (-188.0874, 6.5853) -> (-188.0749, 6.1393)
  line L3236 (-188.0749, 6.1393) -> (-188.111, 5.6946)
  line L3237 (-188.111, 5.6946) -> (-188.1956, 5.2551)
  line L3238 (-188.1956, 5.2551) -> (-188.3053, 4.9274)
  line L3239 (-188.3053, 4.9274) -> (-188.4537, 4.6198)
  line L3240 (-188.4537, 4.6198) -> (-188.6379, 4.3353)
  line L3241 (-188.6379, 4.3353) -> (-188.8553, 4.0767)
  line L3242 (-188.8553, 4.0767) -> (-189.103, 3.8471)
  line L3243 (-189.103, 3.8471) -> (-189.3783, 3.6492)
  line L3244 (-189.3783, 3.6492) -> (-189.6783, 3.4861)
  line L3245 (-189.6783, 3.4861) -> (-190.0003, 3.3606)
  line L3246 (-190.0003, 3.3606) -> (-190.3447, 3.2656)
  line L3247 (-190.3447, 3.2656) -> (-190.6949, 3.1986)
  line L3248 (-190.6949, 3.1986) -> (-191.0495, 3.1599)
  line L3249 (-191.0495, 3.1599) -> (-191.4065, 3.1497)
  line L3250 (-191.4065, 3.1497) -> (-191.7751, 3.1606)
  line L3251 (-191.7751, 3.1606) -> (-192.1412, 3.1995)
  line L3252 (-192.1412, 3.1995) -> (-192.5033, 3.2663)
  line L3253 (-192.5033, 3.2663) -> (-192.8597, 3.3606)
  line L3254 (-192.8597, 3.3606) -> (-193.1496, 3.4694)
  line L3255 (-193.1496, 3.4694) -> (-193.4237, 3.6077)
  line L3256 (-193.4237, 3.6077) -> (-193.6798, 3.7739)
  line L3257 (-193.6798, 3.7739) -> (-193.9159, 3.966)
  line L3258 (-193.9159, 3.966) -> (-194.1301, 4.1823)
  line L3259 (-194.1301, 4.1823) -> (-194.3205, 4.421)
  line L3260 (-194.3205, 4.421) -> (-194.4849, 4.6803)
  line L3261 (-194.4849, 4.6803) -> (-194.6214, 4.9583)
  line L3262 (-194.6214, 4.9583) -> (-194.7415, 5.3308)
  line L3263 (-194.7415, 5.3308) -> (-194.8171, 5.7134)
  line L3264 (-194.8171, 5.7134) -> (-194.8476, 6.1023)
  line L3265 (-194.8476, 6.1023) -> (-194.8323, 6.4934)
  line L3266 (-194.8323, -30.6316) -> (-194.7794, -30.2577)
  line L3267 (-194.7794, -30.2577) -> (-194.6772, -29.8998)
  line L3268 (-194.6772, -29.8998) -> (-194.5286, -29.5619)
  line L3269 (-194.5286, -29.5619) -> (-194.3367, -29.2485)
  line L3270 (-194.3367, -29.2485) -> (-194.1044, -28.9636)
  line L3271 (-194.1044, -28.9636) -> (-193.8348, -28.7116)
  line L3272 (-193.8348, -28.7116) -> (-193.5309, -28.4967)
  line L3273 (-193.5309, -28.4967) -> (-193.1956, -28.323)
  line L3274 (-193.1956, -28.323) -> (-192.8739, -28.2011)
  line L3275 (-192.8739, -28.2011) -> (-192.5434, -28.1081)
  line L3276 (-192.5434, -28.1081) -> (-192.2059, -28.0444)
  line L3277 (-192.2059, -28.0444) -> (-191.8636, -28.0105)
  line L3278 (-191.8636, -28.0105) -> (-191.5218, -28.0015)
  line L3279 (-191.5218, -28.0015) -> (-191.18, -28.0066)
  line L3280 (-191.18, -28.0066) -> (-191.18, -32.8386)
  line L3281 (-191.18, -32.8386) -> (-190.8858, -32.8157)
  line L3282 (-190.8858, -32.8157) -> (-190.5963, -32.7634)
  line L3283 (-190.5963, -32.7634) -> (-190.3134, -32.6824)
  line L3284 (-190.3134, -32.6824) -> (-190.0394, -32.573)
  line L3285 (-190.0394, -32.573) -> (-189.8037, -32.4435)
  line L3286 (-189.8037, -32.4435) -> (-189.593, -32.2834)
  line L3287 (-189.593, -32.2834) -> (-189.4095, -32.0965)
  line L3288 (-189.4095, -32.0965) -> (-189.2553, -31.8861)
  line L3289 (-189.2553, -31.8861) -> (-189.1327, -31.6559)
  line L3290 (-189.1327, -31.6559) -> (-189.044, -31.4094)
  line L3291 (-189.044, -31.4094) -> (-188.9913, -31.1501)
  line L3292 (-188.9913, -31.1501) -> (-188.9769, -30.8816)
  line L3293 (-188.9769, -30.8816) -> (-188.9951, -30.5975)
  line L3294 (-188.9951, -30.5975) -> (-189.055, -30.3191)
  line L3295 (-189.055, -30.3191) -> (-189.1523, -30.0736)
  line L3296 (-189.1523, -30.0736) -> (-189.2933, -29.8503)
  line L3297 (-189.2933, -29.8503) -> (-189.4825, -29.6419)
  line L3298 (-189.4825, -29.6419) -> (-189.7034, -29.4675)
  line L3299 (-189.7034, -29.4675) -> (-189.9949, -29.3003)
  line L3300 (-189.9949, -29.3003) -> (-190.305, -29.1707)
  line L3301 (-190.305, -29.1707) -> (-190.1644, -28.0378)
  line L3302 (-190.1644, -28.0378) -> (-189.7198, -28.1853)
  line L3303 (-189.7198, -28.1853) -> (-189.3089, -28.4034)
  line L3304 (-189.3089, -28.4034) -> (-188.94, -28.6868)
  line L3305 (-188.94, -28.6868) -> (-188.6214, -29.03)
  line L3306 (-188.6214, -29.03) -> (-188.4001, -29.3925)
  line L3307 (-188.4001, -29.3925) -> (-188.235, -29.7812)
  line L3308 (-188.235, -29.7812) -> (-188.1283, -30.1899)
  line L3309 (-188.1283, -30.1899) -> (-188.0823, -30.6121)
  line L3310 (-188.0823, -30.6121) -> (-188.0722, -30.9292)
  line L3311 (-188.0722, -30.9292) -> (-188.0878, -31.2456)
  line L3312 (-188.0878, -31.2456) -> (-188.129, -31.5597)
  line L3313 (-188.129, -31.5597) -> (-188.1956, -31.8699)
  line L3314 (-188.1956, -31.8699) -> (-188.3053, -32.1976)
  line L3315 (-188.3053, -32.1976) -> (-188.4537, -32.5052)
  line L3316 (-188.4537, -32.5052) -> (-188.6379, -32.7897)
  line L3317 (-188.6379, -32.7897) -> (-188.8553, -33.0483)
  line L3318 (-188.8553, -33.0483) -> (-189.103, -33.2779)
  line L3319 (-189.103, -33.2779) -> (-189.3783, -33.4758)
  line L3320 (-189.3783, -33.4758) -> (-189.6783, -33.6389)
  line L3321 (-189.6783, -33.6389) -> (-190.0003, -33.7644)
  line L3322 (-190.0003, -33.7644) -> (-190.3447, -33.8594)
  line L3323 (-190.3447, -33.8594) -> (-190.6949, -33.9264)
  line L3324 (-190.6949, -33.9264) -> (-191.0495, -33.9651)
  line L3325 (-191.0495, -33.9651) -> (-191.4065, -33.9753)
  line L3326 (-191.4065, -33.9753) -> (-191.7751, -33.9644)
  line L3327 (-191.7751, -33.9644) -> (-192.1412, -33.9255)
  line L3328 (-192.1412, -33.9255) -> (-192.5033, -33.8587)
  line L3329 (-192.5033, -33.8587) -> (-192.8597, -33.7644)
  line L3330 (-192.8597, -33.7644) -> (-193.1496, -33.6556)
  line L3331 (-193.1496, -33.6556) -> (-193.4237, -33.5173)
  line L3332 (-193.4237, -33.5173) -> (-193.6798, -33.3511)
  line L3333 (-193.6798, -33.3511) -> (-193.9159, -33.159)
  line L3334 (-193.9159, -33.159) -> (-194.1301, -32.9427)
  line L3335 (-194.1301, -32.9427) -> (-194.3205, -32.704)
  line L3336 (-194.3205, -32.704) -> (-194.4849, -32.4448)
  line L3337 (-194.4849, -32.4448) -> (-194.6214, -32.1668)
  line L3338 (-194.6214, -32.1668) -> (-194.7415, -31.7942)
  line L3339 (-194.7415, -31.7942) -> (-194.8171, -31.4116)
  line L3340 (-194.8171, -31.4116) -> (-194.8476, -31.0227)
  line L3341 (-194.8476, -31.0227) -> (-194.8323, -30.6316)
  line L3342 (-194.8362, -19.8464) -> (-194.7998, -19.5087)
  line L3343 (-194.7998, -19.5087) -> (-194.7386, -19.1746)
  line L3344 (-194.7386, -19.1746) -> (-194.6682, -18.9314)
  line L3345 (-194.6682, -18.9314) -> (-194.5711, -18.6985)
  line L3346 (-194.5711, -18.6985) -> (-194.4484, -18.4781)
  line L3347 (-194.4484, -18.4781) -> (-194.3011, -18.2722)
  line L3348 (-194.3011, -18.2722) -> (-194.1565, -18.1315)
  line L3349 (-194.1565, -18.1315) -> (-193.9947, -18.0126)
  line L3350 (-193.9947, -18.0126) -> (-193.8181, -17.9171)
  line L3351 (-193.8181, -17.9171) -> (-193.6292, -17.8464)
  line L3352 (-193.6292, -17.8464) -> (-193.3281, -17.7752)
  line L3353 (-193.3281, -17.7752) -> (-193.0198, -17.7488)
  line L3354 (-193.0198, -17.7488) -> (-192.7094, -17.7363)
  line L3355 (-192.7094, -17.7363) -> (-192.3987, -17.7332)
  line L3356 (-192.3987, -17.7332) -> (-191.1722, -17.7364)
  line L3357 (-191.1722, -17.7364) -> (-189.9456, -17.7253)
  line L3358 (-189.9456, -17.7253) -> (-189.47, -17.7098)
  line L3359 (-189.47, -17.7098) -> (-188.9964, -17.6628)
  line L3360 (-188.9964, -17.6628) -> (-188.7931, -17.6205)
  line L3361 (-188.7931, -17.6205) -> (-188.595, -17.5599)
  line L3362 (-188.595, -17.5599) -> (-188.4032, -17.4814)
  line L3363 (-188.4032, -17.4814) -> (-188.219, -17.3855)
  line L3364 (-188.219, -17.3855) -> (-188.219, -18.5339)
  line L3365 (-188.219, -18.5339) -> (-188.4111, -18.6159)
  line L3366 (-188.4111, -18.6159) -> (-188.6095, -18.6798)
  line L3367 (-188.6095, -18.6798) -> (-188.8128, -18.7256)
  line L3368 (-188.8128, -18.7256) -> (-189.0198, -18.7527)
  line L3369 (-189.0198, -18.7527) -> (-188.6885, -19.1798)
  line L3370 (-188.6885, -19.1798) -> (-188.4104, -19.6433)
  line L3371 (-188.4104, -19.6433) -> (-188.2605, -20.0005)
  line L3372 (-188.2605, -20.0005) -> (-188.1539, -20.3715)
  line L3373 (-188.1539, -20.3715) -> (-188.0916, -20.7524)
  line L3374 (-188.0916, -20.7524) -> (-188.0745, -21.1394)
  line L3375 (-188.0745, -21.1394) -> (-188.0797, -21.4324)
  line L3376 (-188.0797, -21.4324) -> (-188.1155, -21.7224)
  line L3377 (-188.1155, -21.7224) -> (-188.1817, -22.0071)
  line L3378 (-188.1817, -22.0071) -> (-188.2776, -22.2839)
  line L3379 (-188.2776, -22.2839) -> (-188.3982, -22.5217)
  line L3380 (-188.3982, -22.5217) -> (-188.5508, -22.7346)
  line L3381 (-188.5508, -22.7346) -> (-188.7318, -22.9202)
  line L3382 (-188.7318, -22.9202) -> (-188.9373, -23.0761)
  line L3383 (-188.9373, -23.0761) -> (-189.1637, -23.1999)
  line L3384 (-189.1637, -23.1999) -> (-189.407, -23.2892)
  line L3385 (-189.407, -23.2892) -> (-189.6637, -23.3414)
  line L3386 (-189.6637, -23.3414) -> (-189.93, -23.3543)
  line L3387 (-189.93, -23.3543) -> (-190.18, -23.3388)
  line L3388 (-190.18, -23.3388) -> (-190.4221, -23.2897)
  line L3389 (-190.4221, -23.2897) -> (-190.6531, -23.2088)
  line L3390 (-190.6531, -23.2088) -> (-190.8702, -23.0979)
  line L3391 (-190.8702, -23.0979) -> (-191.0703, -22.9587)
  line L3392 (-191.0703, -22.9587) -> (-191.2505, -22.793)
  line L3393 (-191.2505, -22.793) -> (-191.4079, -22.6027)
  line L3394 (-191.4079, -22.6027) -> (-191.5394, -22.3894)
  line L3395 (-191.5394, -22.3894) -> (-191.6579, -22.1478)
  line L3396 (-191.6579, -22.1478) -> (-191.7537, -21.8969)
  line L3397 (-191.7537, -21.8969) -> (-191.8264, -21.6384)
  line L3398 (-191.8264, -21.6384) -> (-191.8753, -21.3738)
  line L3399 (-191.8753, -21.3738) -> (-191.9924, -20.511)
  line L3400 (-191.9924, -20.511) -> (-192.1292, -19.6511)
  line L3401 (-192.1292, -19.6511) -> (-192.2157, -19.245)
  line L3402 (-192.2157, -19.245) -> (-192.3323, -18.8464)
  line L3403 (-192.3323, -18.8464) -> (-192.765, -18.8455)
  line L3404 (-192.765, -18.8455) -> (-193.1917, -18.9168)
  line L3405 (-193.1917, -18.9168) -> (-193.3611, -18.9885)
  line L3406 (-193.3611, -18.9885) -> (-193.5099, -19.0933)
  line L3407 (-193.5099, -19.0933) -> (-193.6334, -19.227)
  line L3408 (-193.6334, -19.227) -> (-193.7269, -19.3855)
  line L3409 (-193.7269, -19.3855) -> (-193.8115, -19.5803)
  line L3410 (-193.8115, -19.5803) -> (-193.8746, -19.7825)
  line L3411 (-193.8746, -19.7825) -> (-193.9155, -19.9903)
  line L3412 (-193.9155, -19.9903) -> (-193.9339, -20.2019)
  line L3413 (-193.9339, -20.2019) -> (-193.9327, -20.6416)
  line L3414 (-193.9327, -20.6416) -> (-193.8714, -21.0769)
  line L3415 (-193.8714, -21.0769) -> (-193.7854, -21.3347)
  line L3416 (-193.7854, -21.3347) -> (-193.6683, -21.5457)
  line L3417 (-193.6683, -21.5457) -> (-193.5042, -21.7175)
  line L3418 (-193.5042, -21.7175) -> (-193.2894, -21.866)
  line L3419 (-193.2894, -21.866) -> (-193.0039, -21.9987)
  line L3420 (-193.0039, -21.9987) -> (-192.7034, -22.0925)
  line L3421 (-192.7034, -22.0925) -> (-192.8519, -23.1668)
  line L3422 (-192.8519, -23.1668) -> (-193.0831, -23.1123)
  line L3423 (-193.0831, -23.1123) -> (-193.3087, -23.0392)
  line L3424 (-193.3087, -23.0392) -> (-193.5276, -22.9478)
  line L3425 (-193.5276, -22.9478) -> (-193.7386, -22.8386)